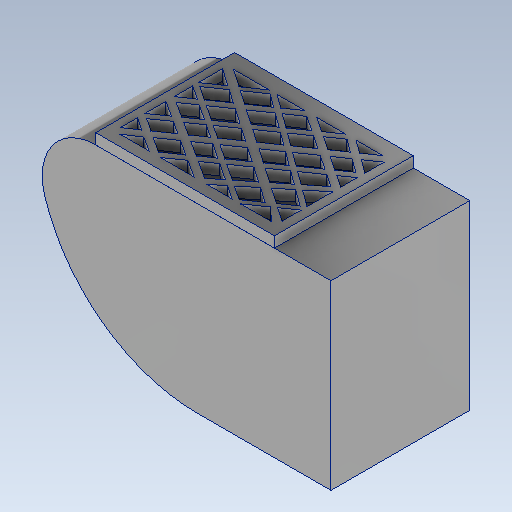
# Autodesk Inventor part: Finray_9_Kerbe_10deg_anschluss_erweitert_9_75 Nut
Saved by Autodesk Inventor 2025.2 (Build 292293000, 293)
## iProperties
Created: 2022-02-28
Part Number: Finray_9_Kerbe_10deg_anschluss_erweitert_9_75 Nut
Material: Generic
Document SubType Name: Modeling
Designer: richa
Density: 1 g/cm^3
Appearance: Aluminum - Flat
Author: richa
## iProperties of the stored document Maria_Greifer_3D-Druck.ipt
Created: 2024-11-10
Part Number: Maria_Greifer_3D-Druck
Material: Generisch
Document SubType Name: Modeling
Designer: maria
Density: 1 g/cm^3
Appearance: Vorgabe
Author: maria
Autodesk Inventor part; units mm, degrees
ref_plane "YZ Plane" through (0, 0, 0) normal (1, 0, 0) x (0, 1, 0)
ref_plane "XZ Plane" through (0, 0, 0) normal (0, 1, 0) x (-1, 0, 0)
ref_plane "XY Plane" through (0, 0, 0) normal (0, 0, 1) x (1, 0, 0)
sketch "Sketch5" plane through (0, 0, 0) normal (0, 0, 1) x (1, 0, 0)
  line L0 (27.5, -17) -> (0, -17)
  line L1 (0, -17) -> (0, 0)
  line L2 (0, 0) -> (7.8, 0)
  line L3 (7.8, 0) -> (27.5, 0)
  line L4 (27.5, 0) -> (27.5, -17)
  dimension "d97" = 17
  dimension "d106" = 27.5
  constraints: 10 end point, 2 horizontal, 2 perpendicular, 1 parallel
  measures "d97" distance of L0.end L1.end
  measures "d106" distance of L0.start L0.end
extrude "Extrusion2" add sketch "Sketch5" along normal blind 13
fillet "Fillet2" radius 15 1 edges at (0, -17, 6.5)
sketch "Sketch11" plane through (0, 0, 13) normal (0, 0, 1) x (1, 0, 0)
  line L0 (44, -2.975) -> (50, -2.975) projected
  circle A0 centre (44, -2.975) radius 0.5
  line L1 (44, -12.625) -> (44, -2.975) projected
  circle A1 centre (44, -12.625) radius 0.5
  line L2 (50, -12.625) -> (44, -12.625) projected
  circle A2 centre (50, -12.625) radius 0.5
  line L3 (50, -2.975) -> (50, -5) projected
  circle A3 centre (50, -2.975) radius 0.5
  point P0 (0, 0)
  dimension "d99" = 1
  dimension "d100" = 1
  dimension "d101" = 1
  dimension "d102" = 1
  constraints: 4 centre point, 1 coincident
  measures "d99" diameter of A0
  measures "d100" diameter of A1
  measures "d101" diameter of A2
  measures "d102" diameter of A3
extrude "Extrusion7" cut sketch "Sketch11" against normal through all
fillet "Rundung3" radius 5 1 edges at (0, 0, 6.5)
sketch "Skizze12" plane through (27.5, 0, 13) normal (0, 1, 0) x (1, 0, 0)
  line L0 (-5.2906, -0.0042) -> (-22.0235, -0.0042)
  line L1 (-22.0235, -0.0042) -> (-5.2906, -0.0042)
  line L2 (-5.2906, 12.9986) -> (-5.2906, -0.0042)
  line L3 (-5.2906, 12.9986) -> (-22.0235, 12.9986)
  line L4 (-22.0235, 12.9986) -> (-22.0235, -0.0042)
  line L5 (-21.2812, 3.1698) -> (-20.0885, 2.3768)
  line L6 (-20.7795, 3.5201) -> (-19.5831, 2.7248)
  line L7 (-18.9333, 2.2927) -> (-17.5217, 1.3544)
  line L8 (-21.2812, 1.5555) -> (-20.0885, 2.3768)
  line L9 (-21.2812, 5.8168) -> (-19.8195, 4.8743)
  line L10 (-20.7049, 6.2136) -> (-19.2473, 5.2738)
  line L11 (-21.2812, 3.8537) -> (-19.8195, 4.8743)
  line L12 (-20.7795, 3.5201) -> (-19.3102, 4.5459)
  line L13 (-21.2812, 8.3321) -> (-19.9905, 7.474)
  line L14 (-19.6031, 7.7408) -> (-20.8965, 8.6007)
  line L15 (-20.7049, 6.2136) -> (-19.4227, 7.0965)
  line L16 (-19.3102, 4.5459) -> (-18.0854, 3.7562)
  line L17 (-17.4257, 3.3308) -> (-18.9333, 2.2927)
  line L18 (-19.5831, 2.7248) -> (-18.0854, 3.7562)
  line L19 (-18.738, 4.9454) -> (-17.509, 4.153)
  line L20 (-19.4227, 7.0965) -> (-17.9955, 6.1477)
  line L21 (-17.6108, 6.4163) -> (-19.0353, 7.3633)
  line L22 (-19.2473, 5.2738) -> (-17.9955, 6.1477)
  line L23 (-18.738, 4.9454) -> (-17.4938, 5.8142)
  line L24 (-19.0353, 7.3633) -> (-17.4312, 8.4679)
  line L25 (-20.8047, 1.004) -> (-18.0235, 1.004)
  line L26 (-16.9948, 1.004) -> (-13.8169, 1.004)
  line L27 (-11.5614, 1.8703) -> (-10.2584, 1.004)
  line L28 (-9.8737, 1.2726) -> (-11.207, 2.159)
  line L29 (-13.2245, 1.3905) -> (-12.1396, 2.2547)
  line L30 (-9.8737, 1.2726) -> (-8.4375, 2.2754)
  line L31 (-7.8193, 2.707) -> (-6.5161, 3.6169)
  line L32 (-7.4222, 2.4336) -> (-6.1314, 3.3348)
  line L33 (-11.7808, 2.5405) -> (-10.4092, 3.633)
  line L34 (-12.6251, 1.004) -> (-11.5614, 1.8703)
  line L35 (-11.207, 2.159) -> (-9.8608, 3.2554)
  line L36 (-8.4375, 2.2754) -> (-9.8608, 3.2554)
  line L37 (-6.1314, 1.5448) -> (-7.4222, 2.4336)
  line L38 (-12.6251, 1.004) -> (-10.2584, 1.004)
  line L39 (-9.4696, 1.004) -> (-6.5911, 1.004)
  line L40 (-6.1314, 1.5448) -> (-6.1314, 3.3348)
  line L41 (-9.2905, 3.7199) -> (-8.0426, 4.7363)
  line L42 (-7.6868, 5.0261) -> (-6.1314, 6.2929)
  line L43 (-9.832, 4.0928) -> (-8.5537, 5.111)
  line L44 (-8.1937, 5.3978) -> (-6.6412, 6.6344)
  line L45 (-8.0426, 4.7363) -> (-6.5161, 3.6169)
  line L46 (-7.6868, 5.0261) -> (-6.1314, 3.8855)
  line L47 (-7.8193, 2.707) -> (-9.2905, 3.7199)
  line L48 (-10.4092, 3.633) -> (-11.8291, 4.6107)
  line L49 (-9.832, 4.0928) -> (-11.211, 5.0423)
  line L50 (-9.8018, 6.0262) -> (-8.5537, 5.111)
  line L51 (-11.7289, 5.3989) -> (-10.3035, 6.3941)
  line L52 (-11.211, 5.0423) -> (-9.8018, 6.0262)
  line L53 (-9.4171, 6.2948) -> (-8.1937, 5.3978)
  line L54 (-6.1314, 3.8855) -> (-6.1314, 6.2929)
  line L55 (-9.4171, 6.2948) -> (-7.8095, 7.4172)
  line L56 (-7.2631, 7.7987) -> (-6.1314, 8.5889)
  line L57 (-7.8095, 7.4172) -> (-6.6412, 6.6344)
  line L58 (-9.9188, 6.6627) -> (-8.3345, 7.7689)
  line L59 (-7.788, 8.1505) -> (-6.6331, 8.9568)
  line L60 (-7.2631, 7.7987) -> (-6.1314, 7.0405)
  line L61 (-6.1314, 7.0405) -> (-6.1314, 8.5889)
  line L62 (-6.1314, 9.3071) -> (-6.1314, 11.1082)
  line L63 (-6.1314, 11.1082) -> (-7.398, 10.2359)
  line L64 (-8.0166, 10.6895) -> (-6.721, 11.5817)
  line L65 (-9.735, 11.2313) -> (-8.5218, 10.3417)
  line L66 (-7.9032, 9.8881) -> (-6.6331, 8.9568)
  line L67 (-9.2333, 11.5817) -> (-8.0166, 10.6895)
  line L68 (-7.398, 10.2359) -> (-6.1314, 9.3071)
  line L69 (-12.9093, 11.5817) -> (-11.5333, 10.6597)
  line L70 (-13.4597, 11.2027) -> (-12.0797, 10.2782)
  line L71 (-11.0334, 10.3248) -> (-9.735, 11.2313)
  line L72 (-11.5333, 10.6597) -> (-10.2128, 11.5817)
  line L73 (-9.7728, 9.4802) -> (-8.5218, 10.3417)
  line L74 (-7.9032, 9.8881) -> (-9.1254, 9.0465)
  line L75 (-11.5799, 9.9433) -> (-10.3231, 9.1013)
  line L76 (-9.6757, 8.6675) -> (-8.3345, 7.7689)
  line L77 (-11.0334, 10.3248) -> (-9.7728, 9.4802)
  line L78 (-9.1254, 9.0465) -> (-7.788, 8.1505)
  line L79 (-11.211, 7.6103) -> (-9.9188, 6.6627)
  line L80 (-11.5983, 7.3436) -> (-10.3035, 6.3941)
  line L81 (-9.6757, 8.6675) -> (-11.211, 7.6103)
  line L82 (-11.8296, 8.0639) -> (-10.3231, 9.1013)
  line L83 (-17.6108, 6.4163) -> (-16.0422, 7.5116)
  line L84 (-17.1091, 6.0828) -> (-15.549, 7.172)
  line L85 (-16.0422, 7.5116) -> (-17.4312, 8.4679)
  line L86 (-15.424, 7.9432) -> (-16.8087, 8.8966)
  line L87 (-13.4054, 8.6687) -> (-12.2169, 7.7972)
  line L88 (-15.424, 7.9432) -> (-13.8832, 9.019)
  line L89 (-13.4985, 9.2876) -> (-12.0797, 10.2782)
  line L90 (-14.9308, 7.6036) -> (-13.4054, 8.6687)
  line L91 (-13.0207, 8.9373) -> (-11.5799, 9.9433)
  line L92 (-13.0207, 8.9373) -> (-11.8296, 8.0639)
  line L93 (-16.8087, 8.8966) -> (-15.2139, 9.9948)
  line L94 (-14.8266, 10.2615) -> (-13.4597, 11.2027)
  line L95 (-17.0117, 11.3131) -> (-15.7543, 10.3911)
  line L96 (-15.2139, 9.9948) -> (-13.8832, 9.019)
  line L97 (-17.3667, 9.2808) -> (-15.7543, 10.3911)
  line L98 (-15.367, 10.6578) -> (-14.0253, 11.5817)
  line L99 (-16.627, 11.5817) -> (-15.367, 10.6578)
  line L100 (-14.8266, 10.2615) -> (-13.4985, 9.2876)
  line L101 (-14.0253, 11.5817) -> (-16.627, 11.5817)
  line L102 (-17.378, 11.5817) -> (-20.7083, 11.5817)
  line L103 (-17.3667, 9.2808) -> (-18.6534, 10.1668)
  line L104 (-19.0316, 10.4271) -> (-20.7083, 11.5817)
  line L105 (-20.8965, 8.6007) -> (-19.2716, 9.7352)
  line L106 (-18.6534, 10.1668) -> (-17.0117, 11.3131)
  line L107 (-21.2812, 8.8564) -> (-19.6497, 9.9955)
  line L108 (-19.0316, 10.4271) -> (-17.378, 11.5817)
  line L109 (-17.9892, 8.8521) -> (-19.2716, 9.7352)
  line L110 (-19.6497, 9.9955) -> (-21.2812, 11.1189)
  line L111 (-21.2812, 11.1189) -> (-21.2812, 8.8564)
  line L112 (-21.2812, 8.3321) -> (-21.2812, 6.5852)
  line L113 (-21.2812, 5.8168) -> (-21.2812, 3.8537)
  line L114 (-21.2812, 3.1698) -> (-21.2812, 1.5555)
  line L115 (-13.8514, 3.917) -> (-12.3471, 4.9673)
  line L116 (-13.7091, 3.2981) -> (-12.1396, 2.2547)
  line L117 (-13.3244, 3.5667) -> (-11.8291, 4.6107)
  line L118 (-11.7808, 2.5405) -> (-13.3244, 3.5667)
  line L119 (-16.8494, 3.7277) -> (-15.4317, 2.8136)
  line L120 (-14.8969, 2.4688) -> (-13.2245, 1.3905)
  line L121 (-17.4257, 3.3308) -> (-16.0039, 2.4141)
  line L122 (-16.9948, 1.004) -> (-15.4691, 2.0693)
  line L123 (-14.8969, 2.4688) -> (-13.7091, 3.2981)
  line L124 (-17.5217, 1.3544) -> (-16.0039, 2.4141)
  line L125 (-15.4317, 2.8136) -> (-14.2361, 3.6484)
  line L126 (-12.3471, 4.9673) -> (-13.6982, 5.8976)
  line L127 (-14.3369, 6.3374) -> (-15.549, 7.172)
  line L128 (-11.5983, 7.3436) -> (-13.0757, 6.3263)
  line L129 (-11.7289, 5.3989) -> (-13.0757, 6.3263)
  line L130 (-13.7144, 6.766) -> (-14.9308, 7.6036)
  line L131 (-13.7144, 6.766) -> (-12.2169, 7.7972)
  line L132 (-13.8514, 3.917) -> (-15.2368, 4.8381)
  line L133 (-15.8867, 5.2702) -> (-17.1091, 6.0828)
  line L134 (-17.4938, 5.8142) -> (-16.2742, 5.0034)
  line L135 (-15.6243, 4.5713) -> (-14.2361, 3.6484)
  line L136 (-13.6982, 5.8976) -> (-15.2368, 4.8381)
  line L137 (-15.6243, 4.5713) -> (-16.8494, 3.7277)
  line L138 (-17.509, 4.153) -> (-16.2742, 5.0034)
  line L139 (-15.8867, 5.2702) -> (-14.3369, 6.3374)
  line L140 (-6.721, 11.5817) -> (-9.2333, 11.5817)
  line L141 (-10.2128, 11.5817) -> (-12.9093, 11.5817)
  line L142 (-13.8169, 1.004) -> (-15.4691, 2.0693)
  line L143 (-21.2812, 6.5852) -> (-19.9905, 7.474)
  line L144 (-19.6031, 7.7408) -> (-17.9892, 8.8521)
  line L145 (-9.4696, 1.004) -> (-7.8095, 2.159)
  line L146 (-7.8095, 2.159) -> (-6.5911, 1.004)
  line L147 (-20.8047, 1.004) -> (-19.4065, 1.8842)
  line L148 (-19.4065, 1.8842) -> (-18.0235, 1.004)
  point P0 (-27.5, 13)
  constraints: 402 parallel, 298 end point, 33 perpendicular, 5 horizontal, 2 point on line
extrude "Extrusion8" add sketch "Skizze12" along normal blind 1
equation "\"l1\" = 8"
body "Solid2"
